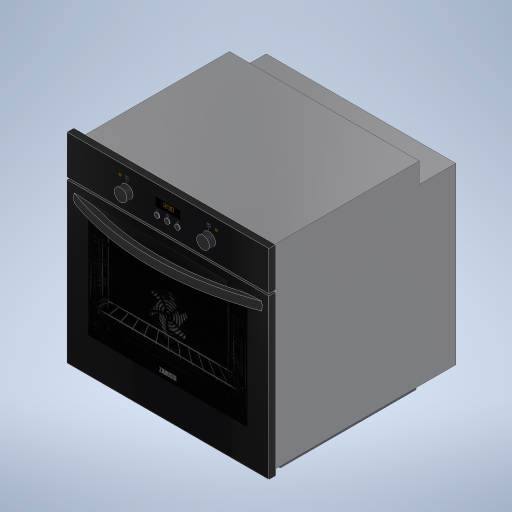
# Autodesk Inventor part: ZANUSI ZOB-35712BK
Saved by Autodesk Inventor 2024 (Build 280153000, 153)
## iProperties
Created: 2015-05-22
Part Number: ZANUSI ZOB-35712BK
Material: Generic
Document SubType Name: Modeling
Designer: SauliusD
Density: 1 g/cm^3
Appearance: Default
Description: ZANUSSI Owen
Author: SauliusD
Autodesk Inventor part; units mm, degrees
ref_plane "YZ Plane" through (0, 0, 0) normal (1, 0, 0) x (0, 1, 0)
ref_plane "XZ Plane" through (0, 0, 0) normal (0, 1, 0) x (-1, 0, 0)
ref_plane "XY Plane" through (0, 0, 0) normal (0, 0, 1) x (1, 0, 0)
sketch "Sketch1" plane through (0, 0, 0) normal (0, 0, 1) x (1, 0, 0)
  line L0 (279, 274) -> (-279, 274)
  line L1 (-279, 274) -> (-279, -274)
  line L2 (-279, -274) -> (279, -274)
  line L3 (279, -274) -> (279, 274)
  line L4 (279, 274) -> (-279, -274) construction
  line L5 (-279, 274) -> (279, -274) construction
  point P0 (0, 0)
  dimension "d0" = 558
  dimension "d1" = 548
  constraints: 12 end point, 2 midpoint, 2 parallel, 1 horizontal, 1 perpendicular
  measures "d0" distance of L2.end L1.end
  measures "d1" distance of L1.end L0.end
extrude "Extrusion1" add sketch "Sketch1" along normal blind 573
sketch "Sketch2" plane through (-279, -274, 0) normal (0, -1, 0) x (1, 0, 0)
  line L0 (-18, 589) -> (576, 589)
  line L1 (576, 589) -> (576, 0)
  line L2 (576, 0) -> (-18, 0)
  line L3 (-18, 0) -> (-18, 589)
  line L4 (0, 0) -> (558, 0) projected
  point P0 (279, 0)
  point P1 (279, 0)
  point P2 (279, 0)
  dimension "d4" = 594
  dimension "d5" = 589
  constraints: 8 end point, 2 midpoint, 2 parallel, 1 coincident, 1 collinear, 1 horizontal, 1 perpendicular
  measures "d4" distance of L0.start L0.end
  measures "d5" distance of L0.end L1.end
extrude "Extrusion2" add sketch "Sketch2" along normal blind 20 separate body
sketch "Sketch3" plane through (-279, -274, 0) normal (-1, 0, 0) x (0, 0, 1)
  line L0 (573, 548) -> (513, 548)
  line L1 (513, 548) -> (513, 440)
  line L2 (513, 440) -> (573, 440)
  line L3 (573, 440) -> (573, 548)
  line L4 (0, 0) -> (573, 0) projected
  line L5 (573, 548) -> (573, 0) projected
  line L6 (0, 548) -> (573, 548) projected
  point P0 (0, 274)
  dimension "d11" = 440
  dimension "d12" = 60
  constraints: 8 end point, 2 collinear, 2 parallel, 1 horizontal, 1 perpendicular
  measures "d11" distance between parallel lines of L4 L2
  measures "d12" distance of L0.start L0.end
extrude "Extrusion3" cut sketch "Sketch3" against normal through all bodies 1
sketch "Sketch4" plane through (-279, -294, 0) normal (0, -1, 0) x (1, 0, 0)
  line L0 (-18, 589) -> (576, 589) construction
  line L1 (576, 589) -> (576, 473.8739) construction
  line L2 (576, 473.8739) -> (-18, 473.8739) construction
  line L3 (-18, 473.8739) -> (-18, 589) construction
  line L4 (576, 0) -> (576, 589) projected
  point P0 (279, 0)
  constraints: 1 collinear, 2 other
sketch "Sketch5" plane through (-297, -274, 0) normal (-1, 0, 0) x (0, 0, 1)
  line L0 (0, 0) -> (589, 0) projected
  line L1 (473.8739, -20) -> (468.0136, -20)
  line L2 (468.0136, -20) -> (468.0136, 0)
  line L3 (468.0136, 0) -> (473.8739, 0)
  line L4 (473.8739, 0) -> (473.8739, -20)
  point P0 (0, 274)
  constraints: 8 end point, 2 parallel, 1 horizontal, 1 perpendicular, 1 point on line
extrude "Extrusion4" cut sketch "Sketch5" against normal through all bodies 2
sketch "Sketch6" plane through (-279, -294, 0) normal (0, -1, 0) x (1, 0, 0)
  line L0 (-18, 468.0136) -> (576, 468.0136) construction
  line L1 (576, 468.0136) -> (576, 2.3856) construction
  line L2 (576, 2.3856) -> (-18, 2.3856) construction
  line L3 (-18, 2.3856) -> (-18, 468.0136) construction
  line L4 (576, 0) -> (576, 468.0136) projected
  point P0 (279, 0)
  constraints: 1 collinear, 2 other
sketch "Sketch7" plane through (-279, -294, 0) normal (0, -1, 0) x (1, 0, 0)
  circle A0 centre (157.8002, 525.4982) radius 18.5052
  circle A1 centre (247.8765, 510.2623) radius 7.2149
  point P0 (279, 0)
  constraints: 2 centre point
extrude "Extrusion5" add sketch "Sketch7" along normal blind 18 separate body contours A0
extrude "Extrusion6" add sketch "Sketch7" along normal blind 2 separate body contours A1
pattern_linear "Rectangular Pattern1" count 3 spacing 30 along (1, 0, 0) of "Extrusion6" bodies 4
mirror "Mirror1" about plane through (0, 0, 0) normal (1, 0, 0) bodies 3
ref_plane "Work Plane1" through (-297, -294, 444.7636) normal (0, 0, 1) x (1, 0, 0)
sketch "Sketch8" plane through (-297, -294, 444.7636) normal (0, 0, 1) x (1, 0, 0)
  line L0 (594, 0) -> (0, 0) projected
  arc A0 (20, 0) -> (297, -50) centre (297, 742.29) ccw
  line L1 (297, -223.3378) -> (297, 903.228) projected
  line L2 (0, 20) -> (0, 0) projected
  line L3 (0, 0) -> (594, 0) projected
  point P0 (297, 294)
  dimension "d29" = 20
  dimension "d32" = 50
  constraints: 3 point on line, 2 point on circle, 1 centre point
  measures "d29" distance from line of A0.start L2
  measures "d32" distance from line of L0 A0.end
ref_plane "Work Plane2" through (0, -344, 444.7636) normal (1, 0, 0) x (0, 1, 0)
sketch "Sketch9" plane through (0, -344, 444.7636) normal (1, 0, 0) x (0, 1, 0)
  arc A0 (0.5, 12.5) -> (0.5, -12.5) centre (156.5, 0) ccw
  arc A1 (23.1723, 4.3118) -> (0.5, 12.5) centre (2.7267, -16.8172) ccw
  line L0 (0, 0) -> (-18.3203, 0) construction
  arc A2 (0.5, -12.5) -> (23.1723, -4.3118) centre (2.7267, 16.8172) ccw
  arc A3 (23.1723, -4.3118) -> (23.1723, 4.3118) centre (19, 0) ccw
  line L1 (25, 10.6734) -> (25, -7.9058) construction
  point P0 (344, -444.7636)
  dimension "d33" = 25
  dimension "d34" = 25
  dimension "d35" = 6
  dimension "d36" = 0.5
  constraints: 9 point on circle, 4 centre point, 4 end point, 3 symmetric about line, 2 tangent, 1 horizontal, 1 horizontal alignment, 1 vertical, 1 other
  measures "d33" distance from line of L0.start L1
  measures "d34" distance of A0.end A0.start
  measures "d35" radius of A3
  measures "d36" horizontal distance of L0.start A0.start
sweep "Sweep1" add profiles "Sketch9" path "Sketch8" separate body path curves A0
mirror "Mirror2" about plane through (0, -344, 444.7636) normal (1, 0, 0) bodies 5
ref_plane "Work Plane3" through (-279, -294, 0) normal (0, -1, 0) x (1, 0, 0)
split "Split1" plane through (-279, -294, 0) removes the side toward (0, 1, 0) bodies 5
move or copy body "Move2" bodies to move or copy 5 copy no translate (0, 0, -13.25)
decal "Decal1"
decal "Decal2"
sketch "Sketch10" plane through (0, 0, 0) normal (0, 0, -1) x (-1, 0, 0)
  line L0 (279, 274) -> (279, -274) projected
  line L1 (279, -242.2075) -> (231.2034, -242.2075)
  line L2 (231.2034, -242.2075) -> (231.2034, 157.0342)
  line L3 (231.2034, 157.0342) -> (279, 157.0342)
  line L4 (279, 157.0342) -> (279, -242.2075)
  point P0 (0, 0)
  constraints: 8 end point, 2 parallel, 1 horizontal, 1 perpendicular, 1 point on line
extrude "Extrusion7" add sketch "Sketch10" along normal blind 5 separate body
mirror "Mirror3" about plane through (0, 0, 0) normal (1, 0, 0) bodies 6
body "Solid1"
body "Solid2"
body "Solid3"
body "Solid4"
body "Solid5"
body "Solid6"
